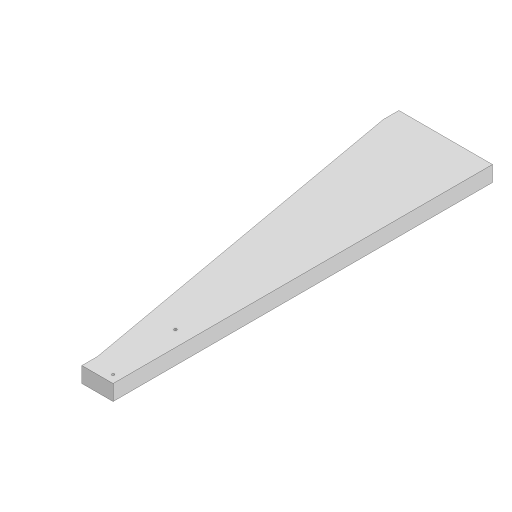
# Autodesk Inventor part: breaker
Saved by Autodesk Inventor 2024 (Build 280153000, 153)
## iProperties
Created: 2024-06-06
Part Number: breaker
Material: 一般
Document SubType Name: Modeling
Designer: USER
Density: 1 g/cm^3
Appearance: 預設
Author: USER
Autodesk Inventor part; units mm, degrees
ref_plane "YZ Plane" through (0, 0, 0) normal (1, 0, 0) x (0, 1, 0)
ref_plane "XZ Plane" through (0, 0, 0) normal (0, 1, 0) x (-1, 0, 0)
ref_plane "XY Plane" through (0, 0, 0) normal (0, 0, 1) x (1, 0, 0)
sketch "草圖1" plane through (0, 0, 0) normal (0, 1, 0) x (-1, 0, 0)
  line L0 (0, 0) -> (6, 0)
  line L1 (6, 0) -> (6, -70)
  line L2 (6, -70) -> (0, -70)
  line L3 (0, -70) -> (0, 0)
  line L4 (0, 0) -> (6, 0)
  line L5 (6, 0) -> (6, 3)
  line L6 (6, 3) -> (0, 3)
  line L7 (0, 3) -> (0, 0)
  line L8 (6, 0) -> (18, -67)
  line L9 (18, -67) -> (18, -70)
  line L10 (18, -70) -> (6, -70)
  circle A0 centre (1.5, 1.5) radius 0.25
  circle A1 centre (3, -12) radius 0.25
  point P0 (6, 1.5)
  dimension "d0" = 70
  dimension "d1" = 6
  dimension "d2" = 3
  dimension "d5" = 12
  dimension "d6" = 3
  dimension "d7" = 0.5
  dimension "d8" = 0.5
  dimension "d9" = 15
  dimension "d10" = 3
  constraints: 22 end point, 4 parallel, 3 perpendicular, 2 centre point, 2 horizontal, 1 midpoint, 1 vertical, 1 vertical alignment
  measures "d0" distance of L2.end L0.start
  measures "d1" distance of L1.end L2.end
  measures "d2" distance of L6.end L0.start
  measures "d5" distance of L9.end L1.end
  measures "d6" distance of L8.end L9.end
  measures "d7" diameter of A0
  measures "d8" diameter of A1
  measures "d9" vertical distance of L6.end A1.centre
  measures "d10" horizontal distance of L6.end A1.centre
extrude "擠出1" add sketch "草圖1" along normal blind 3
